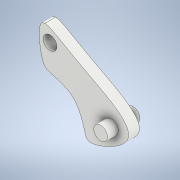
# Autodesk Inventor part: Component20
Saved by Autodesk Inventor 2022 (Build 260153000, 153)
## iProperties
Created: 2022-01-29
Part Number: Component20
Material: Generic
Document SubType Name: Modeling
Designer: Administrator
Density: 1 g/cm^3
Appearance: Default
Title: Component20
Author: Administrator
Autodesk Inventor part; units mm, degrees
ref_plane "YZ Plane" through (0, 0, 0) normal (1, 0, 0) x (0, 1, 0)
ref_plane "XZ Plane" through (0, 0, 0) normal (0, 1, 0) x (-1, 0, 0)
ref_plane "XY Plane" through (0, 0, 0) normal (0, 0, 1) x (1, 0, 0)
sketch "Sketch2" plane through (0, 0, 0) normal (0, 0, 1) x (1, 0, 0)
  circle A0 centre (16.0062, -7.7791) radius 3.175
  circle A1 centre (-12.4507, 11.7346) radius 3.175
  spline S0 degree 5 poles (-14.8456, 18.3233) (-14.2389, 18.3233) (-12.8519, 18.0023) (-10.2839, 16.6995) (-6.1144, 14.2668) (0.0685, 10.7327) (6.8106, 7.2029) (13.6398, 3.634) (19.7273, -0.1328) (24.1069, -4.2799) (24.8345, -8.8077) (20.6824, -13.3013) (14.0153, -17.0348) (7.7478, -19.2304) (4.4145, -19.3007) (3.9747, -17.0166) (2.9128, -12.909) (1.1193, -8.5073) (-1.1175, -5.1358) (-3.2108, -3.4996) (-6.5453, -1.9831) (-10.4668, -0.6946) (-13.6986, 0.0749) (-15.39, 0.9195) (-16.8011, 5.3849) (-17.6987, 11.9046) (-17.4982, 16.416) (-16.4921, 18.0023) (-15.4522, 18.3233) (-14.8456, 18.3233) knots 0 0 0 0 0 0 0.04 0.08 0.12 0.16 0.2 0.24 0.28 0.32 0.36 0.4 0.44 0.48 0.52 0.56 0.6 0.64 0.68 0.72 0.76 0.8 0.84 0.88 0.92 0.96 1 1 1 1 1 1 weights 1 1 1 1 1 1 1 1 1 1 1 1 1 1 1 1 1 1 1 1 1 1 1 1 1 1 1 1 1 1
  point P0 (0, 0)
  constraints: 2 centre point, 1 other
extrude "Extrusion1" add sketch "Sketch2" along normal blind 5 contours A0 | S0
extrude "Extrusion2" add sketch "Sketch2" against normal blind 5 contours A0
sketch "Sketch3" plane through (0, 0, 5) normal (0, 0, 1) x (1, 0, 0)
  circle A0 centre (16.0062, -7.7791) radius 3.175 projected
  circle A1 centre (-12.4507, 11.7346) radius 3.175 projected
  point P0 (0, 0)
  constraints: 1 other
extrude "Extrusion3" add sketch "Sketch3" along normal blind 5 contours A0
body "Solid1"
